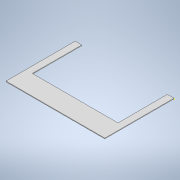
# Autodesk Inventor part: 零件1
Saved by Autodesk Inventor 2022 (Build 260153000, 153)
## iProperties
Created: 2023-03-09
Part Number: 零件1
Material: 一般
Document SubType Name: Modeling
Designer: JOU
Density: 1 g/cm^3
Appearance: 預設
Author: JOU
Autodesk Inventor part; units mm, degrees
ref_plane "YZ Plane" through (0, 0, 0) normal (1, 0, 0) x (0, 1, 0)
ref_plane "XZ Plane" through (0, 0, 0) normal (0, 1, 0) x (-1, 0, 0)
ref_plane "XY Plane" through (0, 0, 0) normal (0, 0, 1) x (1, 0, 0)
sketch "草圖1" plane through (0, 0, 0) normal (0, 1, 0) x (-1, 0, 0)
  point P0 (0, 0)
sketch "草圖2" plane through (0, 0, 0) normal (0, 1, 0) x (-1, 0, 0)
  line L0 (0, 0) -> (300, 0)
  line L1 (300, 0) -> (300, 210)
  line L2 (300, 210) -> (0, 210)
  line L3 (0, 210) -> (0, 0)
  dimension "d0" = 210
  dimension "d1" = 300
  constraints: 8 end point, 2 parallel, 1 horizontal, 1 perpendicular
  measures "d0" distance of L0.end L1.end
  measures "d1" distance of L1.end L2.end
extrude "擠出1" add sketch "草圖2" along normal blind 2
sketch "草圖3" plane through (0, 2, 0) normal (0, 1, 0) x (1, 0, 0)
  line L0 (-280, -150) -> (-20, -150)
  line L1 (-20, -150) -> (-20, 0)
  line L2 (-20, 0) -> (-280, 0)
  line L3 (-280, 0) -> (-280, -150)
  line L4 (0, 0) -> (-300, 0) projected
  line L5 (-300, 0) -> (-300, -210) projected
  dimension "d4" = 260
  dimension "d5" = 150
  dimension "d6" = 20
  constraints: 8 end point, 2 parallel, 1 collinear, 1 horizontal, 1 perpendicular
  measures "d4" distance of L0.start L0.end
  measures "d5" distance of L2.end L0.start
  measures "d6" distance between parallel lines of L5 L3
extrude "擠出2" cut sketch "草圖3" against normal up to surface (2 mm away)
equation "\"d0\" = W_"
equation "\"d1\" = L_"
equation "\"d2\" = h_"
equation "\"d4\" = l_"
equation "\"d5\" = w_"
equation "\"d6\" = -0.5 * l_ + 0.5 * L_"
equation "\"d7\" = h_"
equation "\"W_\" = 210"
equation "\"L_\" = 300"
equation "\"h_\" = 2"
equation "\"w_\" = 150"
equation "\"l_\" = 260"
